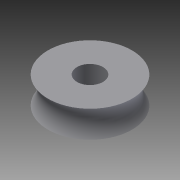
# Autodesk Inventor part: top - top pullet
Saved by Autodesk Inventor 2015 (Build 190159000, 159)
## iProperties
Created: 2014-11-01
Part Number: top - top pullet
Material: Generic
Document SubType Name: Modeling
Designer: jesse
Density: 1 g/cm^3
Appearance: Default
Author: jesse
Autodesk Inventor part; units mm, degrees
ref_plane "YZ Plane" through (0, 0, 0) normal (1, 0, 0) x (0, 1, 0)
ref_plane "XZ Plane" through (0, 0, 0) normal (0, 1, 0) x (-1, 0, 0)
ref_plane "XY Plane" through (0, 0, 0) normal (0, 0, 1) x (1, 0, 0)
sketch "Sketch1" plane through (0, 0, 0) normal (1, 0, 0) x (0, 1, 0)
  line L0 (0, 0) -> (8.128, 0)
  line L1 (8.128, 0) -> (8.128, -12.7)
  line L2 (0, -12.7) -> (0, 0)
  arc A0 (8.128, -12.7) -> (0, -12.7) centre (4.064, -17.8157) ccw
  line L3 (8.128, 0) -> (6.0753, 0)
  line L4 (4.064, 0) -> (4.064, -17.8157) construction
  dimension "d1" = 8.128
  dimension "d2" = 12.7
  constraints: 10 end point, 2 horizontal, 2 point on circle, 1 centre point, 1 midpoint, 1 parallel, 1 perpendicular, 1 vertical
  measures "d1" distance of L0.start L0.end
  measures "d2" distance of L0.end L1.end
revolve "Revolution1" add sketch "Sketch1" angle 360 about axis through (0, 8.128, 0) along (0, -1, 0)
sketch "Sketch2" plane through (0, 0, 0) normal (0, -1, 0) x (1, 0, 0)
  circle A0 centre (0, 0) radius 5.5
  dimension "d3" = 11
  constraints: 1 centre point, 1 coincident
  measures "d3" diameter of A0
extrude "Extrusion1" cut sketch "Sketch2" against normal blind 1.4
sketch "Sketch3" plane through (0, 1.4, 0) normal (0, -1, 0) x (1, 0, 0)
  circle A0 centre (0, 0) radius 3.925
  dimension "d6" = 7.85
  constraints: 1 centre point, 1 coincident
  measures "d6" diameter of A0
extrude "Extrusion2" cut sketch "Sketch3" against normal through all
body "Solid1"
